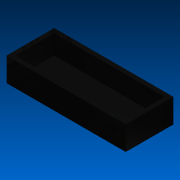
# Autodesk Inventor part: Box
Saved by Autodesk Inventor 2013 (Build 170138000, 138)
## iProperties
Created: 2014-11-03
Part Number: Box
Material: Acetal Resin, Black
Document SubType Name: Modeling
Designer: Jeramy
Density: 1 g/cm^3
Author: Jeramy
Autodesk Inventor part; units mm, degrees
ref_plane "YZ Plane" through (0, 0, 0) normal (1, 0, 0) x (0, 1, 0)
ref_plane "XZ Plane" through (0, 0, 0) normal (0, 1, 0) x (-1, 0, 0)
ref_plane "XY Plane" through (0, 0, 0) normal (0, 0, 1) x (1, 0, 0)
sketch "Sketch4" plane through (0, 0, 0) normal (0, 1, 0) x (-1, 0, 0)
  line L0 (0, 0) -> (-508, 0)
  line L1 (-508, 0) -> (-508, -203.2)
  line L2 (-508, -203.2) -> (0, -203.2)
  line L3 (0, -203.2) -> (0, 0)
  line L4 (0, 0) -> (-19.05, 0)
  dimension "d14" = 508
  dimension "d15" = 203.2
  dimension "d16" = 19.05
  constraints: 10 end point, 2 parallel, 1 horizontal, 1 perpendicular, 1 point on line
  measures "d14" distance of L0.start L0.end
  measures "d15" distance of L0.end L1.end
  measures "d16" distance of L0.start L4.end
extrude "Extrusion3" add sketch "Sketch4" along normal blind 101.6
sketch "Sketch5" plane through (0, 101.6, 0) normal (0, 1, 0) x (1, 0, 0)
  line L0 (0, 0) -> (508, 0) projected
  line L1 (508, 203.2) -> (0, 203.2) projected
  line L2 (0, 0) -> (19.05, 0)
  line L3 (19.05, 19.05) -> (19.05, 184.15)
  line L4 (19.05, 184.15) -> (488.95, 184.15)
  line L5 (488.95, 184.15) -> (488.95, 19.05)
  line L6 (488.95, 19.05) -> (19.05, 19.05)
  dimension "d21" = 165.1
  dimension "d22" = 469.9
  dimension "d23" = 165.1
  constraints: 10 end point, 2 perpendicular, 1 parallel, 1 point on line
  measures "d21" distance of L3.start L3.end
  measures "d22" distance of L3.end L4.end
  measures "d23" distance of L4.end L5.end
extrude "Extrusion4" cut sketch "Sketch5" against normal blind 82.55
fillet "Fillet5" radius 6.35 1 edges at (488.95, 60.325, -184.15)
fillet "Fillet6" radius 6.35 1 edges at (19.05, 60.325, -184.15)
fillet "Fillet7" radius 6.35 1 edges at (19.05, 60.325, -19.05)
fillet "Fillet8" radius 6.35 1 edges at (488.95, 60.325, -19.05)
body "Solid2"
